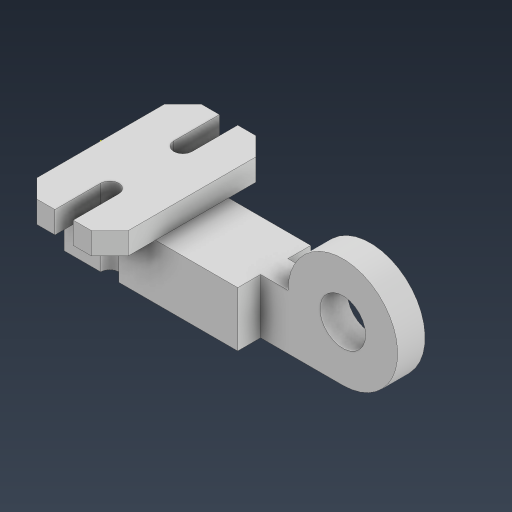
# Autodesk Inventor part: Peça teste 2
Saved by Autodesk Inventor 2024 (Build 280153000, 153)
## iProperties
Created: 2024-02-10
Part Number: Peça teste 2
Material: Genérico
Document SubType Name: Modeling
Designer: Administrator
Density: 1 g/cm^3
Appearance: Padrão
Author: Administrator
Autodesk Inventor part; units mm, degrees
ref_plane "YZ Plane" through (0, 0, 0) normal (1, 0, 0) x (0, 1, 0)
ref_plane "XZ Plane" through (0, 0, 0) normal (0, 1, 0) x (-1, 0, 0)
ref_plane "XY Plane" through (0, 0, 0) normal (0, 0, 1) x (1, 0, 0)
sketch "Esboço1" plane through (0, 0, 0) normal (0, 0, 1) x (1, 0, 0)
  line L0 (0, 0) -> (95, 0)
  line L1 (95, 0) -> (95, 30)
  line L2 (95, 30) -> (0, 30)
  line L3 (0, 30) -> (0, 0)
  line L4 (0, 30) -> (50, 30)
  line L5 (50, 30) -> (50, 42)
  line L6 (50, 42) -> (0, 42)
  line L7 (0, 42) -> (0, 30)
  line L8 (95, 0) -> (140, 0)
  line L9 (110, 30) -> (95, 30)
  line L10 (95, 30) -> (95, 0)
  arc A0 (140, 0) -> (110, 30) centre (140, 30) ccw
  dimension "d0" = 95
  dimension "d1" = 30
  dimension "d2" = 50
  dimension "d3" = 12
  dimension "d4" = 60
  dimension "d5" = 140
  constraints: 22 end point, 5 parallel, 3 horizontal, 2 perpendicular, 2 point on circle, 1 centre point, 1 collinear, 1 tangent
  measures "d0" distance of L2.end L1.end
  measures "d1" distance of L1.end L0.end
  measures "d2" distance of L6.end L5.end
  measures "d3" distance of L5.end L4.end
  measures "d4" diameter of A0
  measures "d5" distance of A0.centre L2.end
extrude "Extrusão1" add sketch "Esboço1" along normal mid plane 40 contours L3 L2 L1 L0
extrude "Extrusão2" add sketch "Esboço1" along normal mid plane 15 contours L1 L9 A0 L8
extrude "Extrusão3" add sketch "Esboço1" along normal mid plane 90 contours L7 L6 L5 L2
sketch "Esboço2" plane through (0, 42, 45) normal (0, 1, 0) x (1, 0, 0)
  point P0 (0, 45)
sketch "Esboço3" plane through (0, 42, 45) normal (0, 1, 0) x (1, 0, 0)
  line L0 (25, -25) -> (25, 25) construction
  line L1 (0, 0) -> (50, 0) projected
  line L2 (30, -25) -> (30, 25)
  line L3 (20, 25) -> (20, -25)
  arc A0 (20, -25) -> (30, -25) centre (25, -25) ccw
  arc A1 (30, 25) -> (20, 25) centre (25, 25) ccw
  line L4 (25, 115) -> (25, 65) construction
  line L5 (50, 90) -> (0, 90) projected
  line L6 (20, 115) -> (20, 65)
  line L7 (30, 65) -> (30, 115)
  arc A2 (30, 115) -> (20, 115) centre (25, 115) ccw
  arc A3 (20, 65) -> (30, 65) centre (25, 65) ccw
  point P0 (0, 45)
  point P1 (25, 0)
  point P2 (25, 90)
  point P3 (30, 90)
  point P4 (20, 90)
  dimension "d12" = 25
  dimension "d14" = 5
  dimension "d15" = 5
  dimension "d16" = 25
  constraints: 16 end point, 8 point on circle, 8 tangent, 4 centre point, 4 midpoint, 2 parallel, 1 perpendicular, 1 vertical
  measures "d12" distance of point (25, 0) L0.end
  measures "d14" radius of A1
  measures "d15" radius of A3
  measures "d16" distance from line of L4.end L5
extrude "Extrusão4" cut sketch "Esboço3" against normal through all contours L3 A1 L2 L1 | L1 L2 A0 L3
extrude "Extrusão5" cut sketch "Esboço3" against normal through all contours L7 A3 L6 L5
chamfer "Chanfro1" distance 10 angle 45 1 edges at (0, 36, 45)
chamfer "Chanfro2" distance 10 angle 45 1 edges at (50, 36, 45)
chamfer "Chanfro3" distance 10 angle 45 2 edges at (0, 36, -45) (50, 36, -45)
sketch "Esboço4" plane through (0, 0, 7.5) normal (0, 0, 1) x (1, 0, 0)
  circle A0 centre (140, 30) radius 12.5
  arc A1 (140, 0) -> (110, 30) centre (140, 30) ccw projected
  point P0 (0, 0)
  dimension "d30" = 25
  constraints: 1 centre point, 1 concentric
  measures "d30" diameter of A0
extrude "Extrusão6" cut sketch "Esboço4" against normal through all
